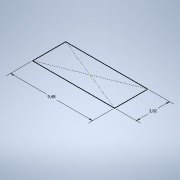
# Autodesk Inventor part: magnet 3.8x9.5
Saved by Autodesk Inventor 2022 (Build 260153000, 153)
## iProperties
Created: 2025-03-24
Part Number: magnet 3.8x9.5
Material: Типовые
Document SubType Name: Modeling
Designer: akap
Density: 1 g/cm^3
Appearance: Титан — полированный
Author: akap
Autodesk Inventor part; units mm, degrees
ref_plane "YZ Plane" through (0, 0, 0) normal (1, 0, 0) x (0, 1, 0)
ref_plane "XZ Plane" through (0, 0, 0) normal (0, 1, 0) x (-1, 0, 0)
ref_plane "XY Plane" through (0, 0, 0) normal (0, 0, 1) x (1, 0, 0)
sketch "Эскиз1" plane through (0, 0, 0) normal (0, 1, 0) x (-1, 0, 0)
  line L0 (4.74, -1.91) -> (-4.74, -1.91)
  line L1 (-4.74, -1.91) -> (-4.74, 1.91)
  line L2 (-4.74, 1.91) -> (4.74, 1.91)
  line L3 (4.74, 1.91) -> (4.74, -1.91)
  line L4 (4.74, -1.91) -> (-4.74, 1.91) construction
  line L5 (-4.74, -1.91) -> (4.74, 1.91) construction
  point P0 (0, 0)
  dimension "d0" = 9.48
  dimension "d1" = 3.82
  constraints: 12 end point, 2 midpoint, 2 parallel, 1 horizontal, 1 perpendicular
  measures "d0" distance of L1.end L2.end
  measures "d1" distance of L0.end L1.end
extrude "Выдавливание1" add sketch "Эскиз1" along normal mid plane 1.73
